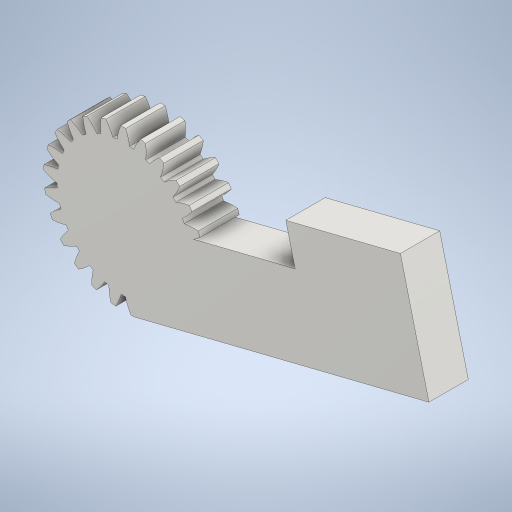
# Autodesk Inventor part: Spur Gear2
Saved by Autodesk Inventor 2024 (Build 280153000, 153)
## iProperties
CustomPartVersion: 1
Created: 2023-09-24
Part Number: Spur Gear2
Material: Steel
Document SubType Name: Modeling
Designer: jebes windows
Categories: <?xml version="1.0" encoding="UTF-16"?> <MemberInstance><Categories><FamilyTemplate><FamilyTemplateParameter ValueType="xs:double" Id="1" ObjectReferenceKey="da_z" ObjectType="kUserParameterObject"/><FamilyTemplateParameter ValueType="xs:double" Id="2" ObjectReferenceKey="da_b" ObjectType="kUserParameterObject"/><FamilyTemplateParameter ValueType="xs:double" Id="3" ObjectReferenceKey="da_beta" ObjectType="kUserParameterObject"/><FamilyTemplateParameter ValueType="xs:double" Id="4" ObjectReferenceKey="da_da" ObjectType="kUserParameterObject"/><FamilyTemplateParameter ValueType="xs:double" Id="5" ObjectReferenceKey="da_aw" ObjectType="kUserParameterObject"/><FamilyTemplateParameter ValueType="xs:string" Id="6" ObjectReferenceKey="EAIAABAAAACIAQAAAAAAAIAAAAAAAAAA" ObjectType="83910656" SubObjectId="SurfaceGeometry"/></FamilyTemplate><ParamToTemplateMap><ParamToTemplate CategoryParameter="//CategoryParameter[@InternalName='046C89C9-8512-4d59-83FE-43B91F4F132A']" TemplateParameter="1"/><ParamToTemplate CategoryParameter="//CategoryParameter[@InternalName='2552DF32-E462-4b46-AEBF-C6C7768E72AC']" TemplateParameter="2"/><ParamToTemplate CategoryParameter="//CategoryParameter[@InternalName='C9EE641D-15FC-4fae-A226-E94C4372FDD7']" TemplateParameter="3"/><ParamToTemplate><ParamToTemplate CategoryParameter="//CategoryParameter[@InternalName='00B6519A-459B-49c7-AD84-2E56D39A5744']" ConstantValue="0.000000"/></ParamToTemplate><ParamToTemplate><ParamToTemplate CategoryParameter="//CategoryParameter[@InternalName='04B31F0E-C7A6-4894-AA32-9629BEFACF47']" ConstantValue="1.000000"/></ParamToTemplate><ParamToTemplate><ParamToTemplate CategoryParameter="//CategoryParameter[@InternalName='43CBEC2E-7847-49e7-A936-2F7889FCB2D9']" ConstantValue="0.250000"/></ParamToTemplate><ParamToTemplate><ParamToTemplate CategoryParameter="//CategoryParameter[@InternalName='B1EFC894-105D-4ebd-86BF-FA20ED196853']" ConstantValue="0.302500"/></ParamToTemplate><ParamToTemplate><ParamToTemplate CategoryParameter="//CategoryParameter[@InternalName='51175063-3D10-4879-93E8-6246FE8B403D']" ConstantValue="2060000000.000000"/></ParamToTemplate><ParamToTemplate><ParamToTemplate CategoryParameter="//CategoryParameter[@InternalName='A3A52E27-4454-46a9-B0BD-C932399B70AF']" ConstantValue="0.300000"/></ParamToTemplate><ParamToTemplate><ParamToTemplate CategoryParameter="//CategoryParameter[@InternalName='91B76062-C214-41d9-B1B9-14D2AB99603D']" ConstantValue="0.100000"/></ParamToTemplate><ParamToTemplate><ParamToTemplate CategoryParameter="//CategoryParameter[@InternalName='374E806E-8B8A-4dda-A9AA-1039D6500AD2']" ConstantValue="10.000000"/></ParamToTemplate><ParamToTemplate><ParamToTemplate CategoryParameter="//CategoryParameter[@InternalName='2D373A89-B862-43d6-8D0B-0CBF12AB9F6C']" ConstantValue="0.349066"/></ParamToTemplate><ParamToTemplate CategoryParameter="//CategoryParameter[@InternalName='37777632-D6A2-4fac-9D53-DB8ACD95C989']" TemplateParameter="4"/><ParamToTemplate CategoryParameter="//CategoryParameter[@InternalName='FD1017F1-B727-4f7e-9707-0F86F1FF9423']" TemplateParameter="5"/><ParamToTemplate><ParamToTemplate CategoryParameter="//CategoryParameter[@InternalName='9E1B4470-B2D3-4ff1-B813-535BB4CDF51A']" ConstantValue="3520000.000000"/></ParamToTemplate><ParamToTemplate><ParamToTemplate CategoryParameter="//CategoryParameter[@InternalName='F8452263-BFF6-458c-9FB1-07C4B99E95CD']" ConstantValue="11400000.000000"/></ParamToTemplate><ParamToTemplate><ParamToTemplate CategoryParameter="//CategoryParameter[@InternalName='3E3BB259-FD49-497f-8171-6EBC954A3479']" ConstantValue="2.000000"/></ParamToTemplate><ParamToTemplate CategoryParameter="//CategoryParameter[@InternalName='27C3BAF2-7550-4e4b-AE2C-0DB134B7D9B7']" TemplateParameter="6"/></ParamToTemplateMap><Category DisplayName="Gear" InternalName="DC85795E-93AB-48d5-8EEE-5A27447B64BD" Mnemonic="Gear"><CategoryParameter DisplayName="z" InternalName="046C89C9-8512-4d59-83FE-43B91F4F132A" Mnemonic="z"/><CategoryParameter DisplayName="b" InternalName="2552DF32-E462-4b46-AEBF-C6C7768E72AC" Mnemonic="b"/><CategoryParameter DisplayName="||b|" InternalName="C9EE641D-15FC-4fae-A226-E94C4372FDD7" Mnemonic="beta"/><CategoryParameter DisplayName="x" InternalName="00B6519A-459B-49c7-AD84-2E56D39A5744" Mnemonic="x"/><CategoryParameter DisplayName="a*" InternalName="04B31F0E-C7A6-4894-AA32-9629BEFACF47" Mnemonic="a"/><CategoryParameter DisplayName="c*" InternalName="43CBEC2E-7847-49e7-A936-2F7889FCB2D9" Mnemonic="c"/><CategoryParameter DisplayName="r|.f|*" InternalName="B1EFC894-105D-4ebd-86BF-FA20ED196853" Mnemonic="rf"/><CategoryParameter DisplayName="E" InternalName="51175063-3D10-4879-93E8-6246FE8B403D" Mnemonic="E"/><CategoryParameter DisplayName="||m|" InternalName="A3A52E27-4454-46a9-B0BD-C932399B70AF" Mnemonic="mi"/><Category DisplayName="SpurGear" InternalName="26C5A22E-A91E-4dfd-A3B3-23CCAFAE1764" Mnemonic="SpurGear"><CategoryParameter DisplayName="m" InternalName="91B76062-C214-41d9-B1B9-14D2AB99603D" Mnemonic="m"/><CategoryParameter DisplayName="P" InternalName="374E806E-8B8A-4dda-A9AA-1039D6500AD2" Mnemonic="PP"/><CategoryParameter DisplayName="||a|" InternalName="2D373A89-B862-43d6-8D0B-0CBF12AB9F6C" Mnemonic="alpha"/><CategoryParameter DisplayName="d|.a|" InternalName="37777632-D6A2-4fac-9D53-DB8ACD95C989" Mnemonic="da"/><CategoryParameter DisplayName="a|.w|" InternalName="FD1017F1-B727-4f7e-9707-0F86F1FF9423" Mnemonic="aw"/><CategoryParameter DisplayName="||s||.Flim|" InternalName="9E1B4470-B2D3-4ff1-B813-535BB4CDF51A" Mnemonic="sFlim"/><CategoryParameter DisplayName="||s||.Hlim|" InternalName="F8452263-BFF6-458c-9FB1-07C4B99E95CD" Mnemonic="sHlim"/><CategoryParameter DisplayName="type" InternalName="3E3BB259-FD49-497f-8171-6EBC954A3479" Mnemonic="type"/><CategoryParameter DisplayName="PitchDiameter" InternalName="27C3BAF2-7550-4e4b-AE2C-0DB134B7D9B7" Mnemonic="IDS_PITCHDIAM"/></Category></Category></Categories></MemberInstance>
Density: 1 g/cm^3
Appearance: Steel
Author: jebes windows
## iProperties of the stored document Spur Gear23_3DPrint.ipt
Created: 2023-09-24
Part Number: Spur Gear23_3DPrint
Material: Generic
Document SubType Name: Modeling
Designer: jebes windows
Density: 1 g/cm^3
Appearance: Default
Author: jebes windows
Autodesk Inventor part; units mm, degrees
sketch "Sketch1" plane through (0, 0, 0) normal (0, 0, 1) x (1, 0, 0)
  circle A0 centre (0, 0) radius 13.5
  dimension "d0" = 27
  constraints: 1 centre point
  measures "d0" diameter of A0
extrude "Extrusion1" add sketch "Sketch1" along normal blind 6.6667
ref_plane "Work Plane2" through (0, 0, 3.3333) normal (0, 0, 1) x (1, 0, 0)
sketch "Sketch2" plane through (0, 0, 0) normal (0, 0, -1) x (-1, 0, 0)
  circle A0 centre (0, 0) radius 13.5 projected
  circle A1 centre (0, 0) radius 12.5
  dimension "d3" = 25
  constraints: 1 centre point, 1 coincident
  measures "d3" diameter of A1
surface extrude "Pitch Diameter" sketch "Sketch2" against normal through all shown no curves A1
ref_plane "Work Plane8" through (0, 0, 0) normal (0.9921147, 0.1253332, 0) x (0, 0, 1)
ref_plane "Work Plane9" through (0, 0, 0) normal (1, 0, 0) x (0, 1, 0)
spur gear teeth "Spur Gear" teeth 25 pitch diameter 25 tip diameter 27 root diameter 22.5 face width 10 start plane through (0, 0, 0) normal (0, 0, -1) x (-1, 0, 0)
sketch "Sketch4" plane through (0, 0, 0) normal (0, 0, -1) x (-1, 0, 0)
  line L0 (-51.7807, -1.0028) -> (-46.9423, 18.4031)
  line L1 (-46.9423, 18.4031) -> (-27.5364, 13.5647)
  arc A0 (3.8108, 10.5849) -> (3.7664, 12.964) centre (-5.3728, 11.6034) ccw projected
  arc A1 (3.7664, 12.964) -> (2.9449, 13.1749) centre (0, 0) ccw projected
  arc A2 (2.9449, 13.1749) -> (1.7599, 11.1115) centre (10.2982, 7.5798) ccw projected
  arc A3 (1.7599, 11.1115) -> (1.0587, 11.2001) centre (0, 0) ccw projected
  arc A4 (1.0587, 11.2001) -> (0.424, 13.4933) centre (-8.0896, 9.9027) ccw projected
  arc A5 (0.424, 13.4933) -> (-0.424, 13.4933) centre (0, 0) ccw projected
  arc A6 (-0.424, 13.4933) -> (-1.0587, 11.2001) centre (8.0896, 9.9027) ccw projected
  arc A7 (-1.0587, 11.2001) -> (-1.7599, 11.1115) centre (0, 0) ccw projected
  arc A8 (-1.7599, 11.1115) -> (-2.9449, 13.1749) centre (-10.2982, 7.5798) ccw projected
  arc A9 (-2.9449, 13.1749) -> (-3.7664, 12.964) centre (0, 0) ccw projected
  arc A10 (-3.7664, 12.964) -> (-3.8108, 10.5849) centre (5.3728, 11.6034) ccw projected
  arc A11 (-3.8108, 10.5849) -> (-4.4679, 10.3247) centre (0, 0) ccw projected
  arc A12 (-4.4679, 10.3247) -> (-6.1289, 12.0286) centre (-11.8596, 4.7806) ccw projected
  arc A13 (-6.1289, 12.0286) -> (-6.8721, 11.62) centre (0, 0) ccw projected
  arc A14 (-6.8721, 11.62) -> (-6.3234, 9.3047) centre (2.3183, 12.575) ccw projected
  arc A15 (-6.3234, 9.3047) -> (-6.8952, 8.8892) centre (0, 0) ccw projected
  arc A16 (-6.8952, 8.8892) -> (-8.9277, 10.1265) centre (-12.6759, 1.681) ccw projected
  arc A17 (-8.9277, 10.1265) -> (-9.5459, 9.5459) centre (0, 0) ccw projected
  arc A18 (-9.5459, 9.5459) -> (-8.4387, 7.4398) centre (-0.8818, 12.7565) ccw projected
  arc A19 (-8.4387, 7.4398) -> (-8.8892, 6.8952) centre (0, 0) ccw projected
  arc A20 (-8.8892, 6.8952) -> (-11.1656, 7.5881) centre (-12.6957, -1.5242) ccw projected
  arc A21 (-11.1656, 7.5881) -> (-11.62, 6.8721) centre (0, 0) ccw projected
  arc A22 (-11.62, 6.8721) -> (-10.0238, 5.1074) centre (-4.0265, 12.1364) ccw projected
  arc A23 (-10.0238, 5.1074) -> (-10.3247, 4.4679) centre (0, 0) ccw projected
  arc A24 (-10.3247, 4.4679) -> (-12.7019, 4.573) centre (-11.9178, -4.6336) ccw projected
  arc A25 (-12.7019, 4.573) -> (-12.964, 3.7664) centre (0, 0) ccw projected
  arc A26 (-12.964, 3.7664) -> (-10.9791, 2.4541) centre (-6.9182, 10.7538) ccw projected
  arc A27 (-10.9791, 2.4541) -> (-11.1115, 1.7599) centre (0, 0) ccw projected
  arc A28 (-11.1115, 1.7599) -> (-13.4401, 1.2705) centre (-10.3911, -7.4519) ccw projected
  arc A29 (-13.4401, 1.2705) -> (-13.4933, 0.424) centre (0, 0) ccw projected
  arc A30 (-13.4933, 0.424) -> (-11.2444, -0.3534) centre (-9.3752, 8.6954) ccw projected
  arc A31 (-11.2444, -0.3534) -> (-11.2001, -1.0587) centre (0, 0) ccw projected
  arc A32 (-11.2001, -1.0587) -> (-13.3338, -2.1119) centre (-8.2114, -9.8019) ccw projected
  arc A33 (-13.3338, -2.1119) -> (-13.1749, -2.9449) centre (0, 0) ccw projected
  arc A34 (-13.1749, -2.9449) -> (-10.8033, -3.1386) centre (-11.2431, 6.0907) ccw projected
  arc A35 (-10.8033, -3.1386) -> (-10.5849, -3.8108) centre (0, 0) ccw projected
  arc A36 (-10.5849, -3.8108) -> (-12.3897, -5.3615) centre (-5.5158, -11.5361) ccw projected
  arc A37 (-12.3897, -5.3615) -> (-12.0286, -6.1289) centre (0, 0) ccw projected
  arc A38 (-12.0286, -6.1289) -> (-9.6833, -5.7267) centre (-12.4046, 3.1033) ccw projected
  arc A39 (-9.6833, -5.7267) -> (-9.3047, -6.3234) centre (0, 0) ccw projected
  arc A40 (-9.3047, -6.3234) -> (-10.6671, -8.2742) centre (-2.4736, -12.5454) ccw projected
  arc A41 (-10.6671, -8.2742) -> (-10.1265, -8.9277) centre (0, 0) ccw projected
  arc A42 (-10.1265, -8.9277) -> (-7.955, -7.955) centre (-12.7867, -0.0791) ccw projected
  arc A43 (-7.955, -7.955) -> (-7.4398, -8.4387) centre (0, 0) ccw projected
  arc A44 (-7.4398, -8.4387) -> (-8.2742, -10.6671) centre (0.724, -12.7664) ccw projected
  arc A45 (-8.2742, -10.6671) -> (-7.5881, -11.1656) centre (0, 0) ccw projected
  arc A46 (-7.5881, -11.1656) -> (-5.7267, -9.6833) centre (-12.3653, -3.2565) ccw projected
  arc A47 (-5.7267, -9.6833) -> (-5.1074, -10.0238) centre (0, 0) ccw projected
  arc A48 (-5.1074, -10.0238) -> (-5.3615, -12.3897) centre (3.8761, -12.1853) ccw projected
  arc A49 (-5.3615, -12.3897) -> (-4.573, -12.7019) centre (0, 0) ccw projected
  arc A50 (-4.573, -12.7019) -> (-3.1386, -10.8033) centre (-11.167, -6.2293) ccw projected
  arc A51 (-3.1386, -10.8033) -> (-2.4541, -10.9791) centre (0, 0) ccw projected
  arc A52 (-2.4541, -10.9791) -> (-2.1119, -13.3338) centre (6.7847, -10.8385) ccw projected
  arc A53 (-2.1119, -13.3338) -> (-1.2705, -13.4401) centre (0, 0) ccw projected
  arc A54 (-1.2705, -13.4401) -> (-0.3534, -11.2444) centre (-9.267, -8.8107) ccw projected
  arc A55 (-0.3534, -11.2444) -> (0.3534, -11.2444) centre (0, 0) ccw projected
  arc A56 (0.3534, -11.2444) -> (1.2705, -13.4401) centre (9.267, -8.8107) ccw projected
  arc A57 (1.2705, -13.4401) -> (2.1119, -13.3338) centre (0, 0) ccw projected
  arc A58 (2.1119, -13.3338) -> (2.4541, -10.9791) centre (-6.7847, -10.8385) ccw projected
  arc A59 (2.4541, -10.9791) -> (3.1386, -10.8033) centre (0, 0) ccw projected
  arc A60 (3.1386, -10.8033) -> (4.573, -12.7019) centre (11.167, -6.2293) ccw projected
  arc A61 (4.573, -12.7019) -> (5.3615, -12.3897) centre (0, 0) ccw projected
  arc A62 (5.3615, -12.3897) -> (5.1074, -10.0238) centre (-3.8761, -12.1853) ccw projected
  arc A63 (5.1074, -10.0238) -> (5.7267, -9.6833) centre (0, 0) ccw projected
  arc A64 (5.7267, -9.6833) -> (7.5881, -11.1656) centre (12.3653, -3.2565) ccw projected
  arc A65 (7.5881, -11.1656) -> (8.2742, -10.6671) centre (0, 0) ccw projected
  arc A66 (8.2742, -10.6671) -> (7.4398, -8.4387) centre (-0.724, -12.7664) ccw projected
  arc A67 (7.4398, -8.4387) -> (7.955, -7.955) centre (0, 0) ccw projected
  arc A68 (7.955, -7.955) -> (10.1265, -8.9277) centre (12.7867, -0.0791) ccw projected
  arc A69 (10.1265, -8.9277) -> (10.6671, -8.2742) centre (0, 0) ccw projected
  arc A70 (10.6671, -8.2742) -> (9.3047, -6.3234) centre (2.4736, -12.5454) ccw projected
  arc A71 (9.3047, -6.3234) -> (9.6833, -5.7267) centre (0, 0) ccw projected
  arc A72 (9.6833, -5.7267) -> (12.0286, -6.1289) centre (12.4046, 3.1033) ccw projected
  arc A73 (12.0286, -6.1289) -> (12.3897, -5.3615) centre (0, 0) ccw projected
  arc A74 (12.3897, -5.3615) -> (10.5849, -3.8108) centre (5.5158, -11.5361) ccw projected
  arc A75 (10.5849, -3.8108) -> (10.8033, -3.1386) centre (0, 0) ccw projected
  arc A76 (10.8033, -3.1386) -> (13.1749, -2.9449) centre (11.2431, 6.0907) ccw projected
  arc A77 (13.1749, -2.9449) -> (13.3338, -2.1119) centre (0, 0) ccw projected
  arc A78 (13.3338, -2.1119) -> (11.2001, -1.0587) centre (8.2114, -9.8019) ccw projected
  arc A79 (11.2001, -1.0587) -> (11.2444, -0.3534) centre (0, 0) ccw projected
  arc A80 (11.2444, -0.3534) -> (13.4933, 0.424) centre (9.3752, 8.6954) ccw projected
  arc A81 (13.4933, 0.424) -> (13.4401, 1.2705) centre (0, 0) ccw projected
  arc A82 (13.4401, 1.2705) -> (11.1115, 1.7599) centre (10.3911, -7.4519) ccw projected
  arc A83 (11.1115, 1.7599) -> (10.9791, 2.4541) centre (0, 0) ccw projected
  arc A84 (10.9791, 2.4541) -> (12.964, 3.7664) centre (6.9182, 10.7538) ccw projected
  arc A85 (12.964, 3.7664) -> (12.7019, 4.573) centre (0, 0) ccw projected
  arc A86 (12.7019, 4.573) -> (10.3247, 4.4679) centre (11.9178, -4.6336) ccw projected
  arc A87 (10.3247, 4.4679) -> (10.0238, 5.1074) centre (0, 0) ccw projected
  arc A88 (10.0238, 5.1074) -> (11.62, 6.8721) centre (4.0265, 12.1364) ccw projected
  arc A89 (11.62, 6.8721) -> (11.1656, 7.5881) centre (0, 0) ccw projected
  arc A90 (11.1656, 7.5881) -> (8.8892, 6.8952) centre (12.6957, -1.5242) ccw projected
  arc A91 (8.8892, 6.8952) -> (8.4387, 7.4398) centre (0, 0) ccw projected
  arc A92 (8.4387, 7.4398) -> (9.5459, 9.5459) centre (0.8818, 12.7565) ccw projected
  arc A93 (9.5459, 9.5459) -> (8.9277, 10.1265) centre (0, 0) ccw projected
  arc A94 (8.9277, 10.1265) -> (6.8952, 8.8892) centre (12.6759, 1.681) ccw projected
  arc A95 (6.8952, 8.8892) -> (6.3234, 9.3047) centre (0, 0) ccw projected
  arc A96 (6.3234, 9.3047) -> (6.8721, 11.62) centre (-2.3183, 12.575) ccw projected
  arc A97 (6.8721, 11.62) -> (6.1289, 12.0286) centre (0, 0) ccw projected
  arc A98 (6.1289, 12.0286) -> (4.4679, 10.3247) centre (11.8596, 4.7806) ccw projected
  arc A99 (4.4679, 10.3247) -> (3.8108, 10.5849) centre (0, 0) ccw projected
  line L2 (0, 0) -> (20.6123, 0) construction
  line L3 (-29.1089, 7.2577) -> (-27.5364, 13.5647)
  line L4 (-29.1089, 7.2577) -> (-22.6088, 7.2577) construction
  line L5 (0, 0) -> (-29.1089, 7.2577)
  line L6 (0, 0) -> (-8.8892, 0)
  line L7 (-51.7807, -1.0028) -> (-1.7807, -13.4692)
  line L8 (-1.7807, -13.4692) -> (-1.2705, -13.4401)
  point P0 (-11.8873, 2.9638)
  dimension "d50" = 20
  dimension "d51" = 20
  dimension "d59" = 76
  dimension "d60" = 6.307
  dimension "d61" = 30
  dimension "d62" = 90
  dimension "d63" = 90
  dimension "d64" = 90
  dimension "d65" = 50
  constraints: 18 end point, 3 horizontal, 1 equal length, 1 perpendicular
  measures "d50" distance of L0.start L0.end
  measures "d51" distance of L1.end L0.end
  measures "d59" angle of L4 L3
  measures "d60" vertical distance of L3.start L1.end
  measures "d61" distance of L2.start L3.start
  measures "d62" angle of L3 L1
  measures "d63" angle of L5 L3
  measures "d64" angle of L0 L7
  measures "d65" horizontal distance of L0.start L7.end
extrude "Extrusion2" add sketch "Sketch4" against normal up to surface (6.6667 mm away) contours L0 L1 L3 L5 A26 A27 A28 A29 A30 A31 A32 A33 A34 A35 A36 A37 A38 A39 A40 A41 A42 A43 A44 A45 A46 A47 A48 A49 A50 A51 A52 A53 L8 L7
equation "\"d0\" = da_da"
equation "\"d1\" = 0.666667 * da_b"
equation "\"d3\" = da_d"
equation "\"d16\" = da_aw"
equation "\"d43\" = da_aw"
equation "\"d46\" = da_aw"
equation "\"da_da\" = 27"
equation "\"da_b\" = 10"
equation "\"da_d\" = 25"
equation "\"da_aw\" = 25"
body "Solid1"
body "Srf1"
